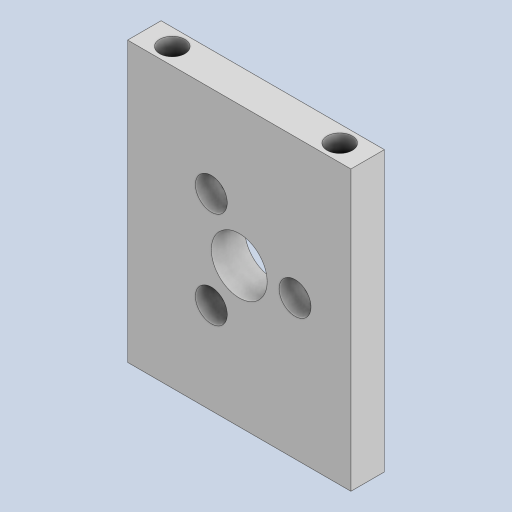
# Autodesk Inventor part: connect-wrist
Saved by Autodesk Inventor 2023 (Build 270158000, 158)
## iProperties
Created: 2024-11-29
Part Number: connect-wrist
Material: Generic
Document SubType Name: Modeling
Designer: kiyo
Density: 1 g/cm^3
Appearance: Default
Author: kiyo
Autodesk Inventor part; units mm, degrees
ref_plane "YZ Plane" through (0, 0, 0) normal (1, 0, 0) x (0, 1, 0)
ref_plane "XZ Plane" through (0, 0, 0) normal (0, 1, 0) x (-1, 0, 0)
ref_plane "XY Plane" through (0, 0, 0) normal (0, 0, 1) x (1, 0, 0)
sketch "スケッチ1" plane through (0, 0, 0) normal (1, 0, 0) x (0, 1, 0)
  line L0 (-20, -25) -> (-20, 25)
  line L1 (-20, 25) -> (20, 25)
  line L2 (20, 25) -> (20, -25)
  line L3 (20, -25) -> (-20, -25)
  line L4 (-20, -25) -> (20, 25) construction
  line L5 (-20, 25) -> (20, -25) construction
  circle A0 centre (0, 0) radius 5
  circle A1 centre (10, 0) radius 1.6
  line L6 (0, 0) -> (18.1986, 0)
  circle A2 centre (10, 0) radius 2.85
  circle A3 centre (-5, 8.6603) radius 2.85
  circle A4 centre (-5, 8.6603) radius 1.6
  circle A5 centre (-5, -8.6603) radius 2.85
  circle A6 centre (-5, -8.6603) radius 1.6
  point P0 (0, 0)
  dimension "d0" = 40
  dimension "d1" = 50
  dimension "d8" = 10
  dimension "d9" = 10
  dimension "d10" = 3.2
  dimension "d11" = 5.7
  dimension "d14" = 360
  constraints: 14 end point, 7 centre point, 4 coincident, 3 midpoint, 2 parallel, 1 horizontal, 1 perpendicular, 1 point on line, 1 vertical, 13 other
  measures "d0" distance of L0.end L1.end
  measures "d1" distance of L1.end L2.end
  measures "d8" diameter of A0
  measures "d9" distance of A1.centre point (0, 0)
  measures "d10" diameter of A1
  measures "d11" diameter of A2
extrude "押し出し1" add sketch "スケッチ1" against normal blind 6 contours L0 L1 L2 L3 | A0 | A2 L6 A1 | L6 A1 A2 | L6 A1 | A1 L6 | A3 | A4 | A5 | A6
extrude "押し出し2" cut sketch "スケッチ1" against normal blind 6 contours A0 | L6 A1 | A1 L6 | A4 | A6
extrude "押し出し3" cut sketch "スケッチ1" against normal blind 4 contours A2 L6 A1 | L6 A1 A2 | A3 | A5
sketch "スケッチ2" plane through (0, -20, 25) normal (0, 0, 1) x (1, 0, 0)
  circle A0 centre (-3, 5) radius 2.25
  circle A1 centre (-3, 35) radius 2.25
  line L0 (-6, 0) -> (-6, 40) projected
  line L1 (0, 0) -> (-6, 0) projected
  line L2 (0, 40) -> (-6, 40) projected
  point P0 (0, 20)
  dimension "d20" = 3
  dimension "d21" = 3
  dimension "d22" = 4.5
  dimension "d23" = 4.5
  dimension "d24" = 5
  dimension "d25" = 5
  constraints: 2 centre point
  measures "d20" distance from line of L0 A0.centre
  measures "d21" distance from line of L0 A1.centre
  measures "d22" diameter of A1
  measures "d23" diameter of A0
  measures "d24" distance from line of L1 A0.centre
  measures "d25" distance from line of L2 A1.centre
extrude "押し出し4" cut sketch "スケッチ2" against normal blind 5
sketch "スケッチ3" plane through (0, -20, -25) normal (0, 0, -1) x (-1, 0, 0)
  circle A0 centre (3, 5) radius 2.25 projected
  circle A1 centre (3, 35) radius 2.25 projected
  circle A2 centre (3, 5) radius 2.25 projected
  circle A3 centre (3, 5) radius 2.25
  circle A4 centre (3, 35) radius 2.25
  point P0 (0, 20)
  constraints: 2 centre point, 2 coincident, 2 concentric
extrude "押し出し5" cut sketch "スケッチ3" against normal blind 5
